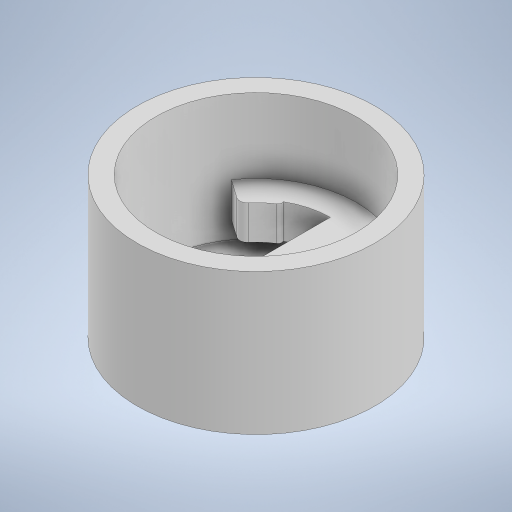
# Autodesk Inventor part: kumi4-2
Saved by Autodesk Inventor 2023.2 (Build 272271000, 271)
## iProperties
Created: 2022-12-20
Part Number: kumi4-2
Material: 一般
Document SubType Name: Modeling
Designer: 千葉 俊輔
Density: 1 g/cm^3
Appearance: 既定
Author: 千葉 俊輔
Autodesk Inventor part; units mm, degrees
ref_plane "YZ Plane" through (0, 0, 0) normal (1, 0, 0) x (0, 1, 0)
ref_plane "XZ Plane" through (0, 0, 0) normal (0, 1, 0) x (-1, 0, 0)
ref_plane "XY Plane" through (0, 0, 0) normal (0, 0, 1) x (1, 0, 0)
sketch "スケッチ1" plane through (0, 0, 0) normal (0, 1, 0) x (-1, 0, 0)
  circle A0 centre (0, 0) radius 16
  dimension "d0" = 32
  constraints: 1 centre point, 1 coincident
  measures "d0" diameter of A0
extrude "押し出し1" add sketch "スケッチ1" along normal blind 2
sketch "スケッチ2" plane through (0, 2, 0) normal (0, 1, 0) x (1, 0, 0)
  circle A0 centre (0, 0) radius 16
  circle A1 centre (0, 0) radius 13.5
  dimension "d3" = 32
  dimension "d4" = 27
  constraints: 2 centre point, 2 coincident
  measures "d3" diameter of A0
  measures "d4" diameter of A1
extrude "押し出し2" add sketch "スケッチ2" along normal blind 17
sketch "スケッチ3" plane through (0, 2, 0) normal (0, 1, 0) x (1, 0, 0)
  arc A0 (-11.0586, -7.7433) -> (0, -13.5) centre (0, 0) ccw
  line L0 (0, 0) -> (-11.0586, -7.7433) construction
  line L1 (0, 0) -> (0, -13.5) construction
  arc A1 (11.0586, 7.7433) -> (0, 13.5) centre (0, 0) ccw
  line L2 (0, 0) -> (11.0586, 7.7433) construction
  line L3 (0, 0) -> (0, 13.5) construction
  circle A2 centre (0, 0) radius 13.5 projected
  line L4 (-11.0586, -7.7433) -> (0, 0)
  line L5 (0, 0) -> (0, -13.5)
  line L6 (0, 13.5) -> (0, 0)
  line L7 (0, 0) -> (11.0586, 7.7433)
  dimension "d7" = 13.5
  dimension "d8" = 55
  dimension "d9" = 13.5
  dimension "d10" = 55
  constraints: 16 end point, 4 point on circle, 2 centre point, 2 coincident, 1 collinear, 1 vertical
  measures "d7" radius of A0
  measures "d8" angle of L0 L1
  measures "d9" radius of A1
  measures "d10" angle of L2 L3
extrude "押し出し3" add sketch "スケッチ3" along normal blind 7 contours L4 L5 A0 | A1 L7 L6
sketch "スケッチ4" plane through (0, 9, 0) normal (0, 1, 0) x (1, 0, 0)
  line L0 (0, -13.5) -> (0, 0) projected
  arc A0 (0, -13.5) -> (11.0586, -7.7433) centre (0, 0) ccw
  line L1 (0, 0) -> (11.0586, -7.7433) construction
  line L2 (0, 0) -> (0, -13.5) construction
  line L3 (0, 0) -> (-11.0586, -7.7433) projected
  arc A1 (0, -10) -> (5, -8.6603) centre (0, 0) ccw
  line L4 (0, 0) -> (5, -8.6603) construction
  line L5 (0, 0) -> (0, -10) construction
  arc A2 (4.75, -8.2272) -> (7.7819, -5.449) centre (0, 0) ccw
  line L6 (0, 0) -> (7.7819, -5.449) construction
  line L7 (0, 0) -> (4.75, -8.2272) construction
  line L8 (0, -13.5) -> (0, -10)
  line L9 (5, -8.6603) -> (4.75, -8.2272)
  line L10 (7.7819, -5.449) -> (11.0586, -7.7433)
  dimension "d13" = 13.5
  dimension "d14" = 55
  dimension "d15" = 10
  dimension "d16" = 30
  dimension "d17" = 9.5
  dimension "d18" = 25
  constraints: 18 end point, 6 point on circle, 3 centre point, 3 coincident, 2 collinear, 1 point on line
  measures "d13" radius of A0
  measures "d14" angle of L2 L1
  measures "d15" radius of A1
  measures "d16" angle of L5 L4
  measures "d17" radius of A2
  measures "d18" angle of L7 L6
sketch "スケッチ5" plane through (0, 9, 0) normal (0, 1, 0) x (1, 0, 0)
  line L0 (0, -13.5) -> (0, 0) projected
  line L1 (0, 13.5) -> (0, 0) projected
  arc A0 (0, 13.5) -> (-11.0586, 7.7433) centre (0, 0) ccw
  line L2 (0, 0) -> (-11.0586, 7.7433) construction
  line L3 (0, 0) -> (0, 13.5) construction
  line L4 (0, 0) -> (-11.0586, -7.7433) projected
  arc A1 (0, 10) -> (-5, 8.6603) centre (0, 0) ccw
  line L5 (0, 0) -> (-5, 8.6603) construction
  line L6 (0, 0) -> (0, 10) construction
  arc A2 (-4.75, 8.2272) -> (-7.7819, 5.449) centre (0, 0) ccw
  line L7 (0, 0) -> (-7.7819, 5.449) construction
  line L8 (0, 0) -> (-4.75, 8.2272) construction
  line L9 (0, 13.5) -> (0, 10)
  line L10 (-5, 8.6603) -> (-4.75, 8.2272)
  line L11 (-11.0586, 7.7433) -> (-7.7819, 5.449)
  dimension "d21" = 13.5
  dimension "d22" = 55
  dimension "d23" = 10
  dimension "d24" = 30
  dimension "d25" = 9.5
  dimension "d26" = 25
  constraints: 18 end point, 6 point on circle, 3 centre point, 3 coincident, 2 collinear, 1 point on line
  measures "d21" radius of A0
  measures "d22" angle of L3 L2
  measures "d23" radius of A1
  measures "d24" angle of L6 L5
  measures "d25" radius of A2
  measures "d26" angle of L8 L7
extrude "押し出し4" add sketch "スケッチ4" against normal blind 4.6
extrude "押し出し5" add sketch "スケッチ5" against normal blind 4.6
fillet "フィレット1" radius 1 2 edges at (-7.7819, 6.7, -5.449) (7.7819, 6.7, 5.449)
fillet "フィレット2" radius 0.5 1 edges at (-4.75, 6.7, -8.2272)
fillet "フィレット3" radius 0.5 1 edges at (4.75, 6.7, 8.2272)
